fc_esc_stack_20x20mm (Autodesk Fusion 360 design; units mm, degrees)
Autodesk Fusion 360 part; units mm, degrees
sketch "Sketch1" plane through (0, 0, 0) normal (0, 1, 0) x (1, 0, 0)
  line L0 (13.5, -13.5) -> (-13.5, -13.5)
  line L1 (-13.5, -13.5) -> (-13.5, 13.5)
  line L2 (-13.5, 13.5) -> (13.5, 13.5)
  line L3 (13.5, 13.5) -> (13.5, -13.5)
  line L4 (13.5, -13.5) -> (-13.5, 13.5) construction
  line L5 (-13.5, -13.5) -> (13.5, 13.5) construction
  circle A0 centre (10, -10) radius 1.5
  circle A1 centre (-10, -10) radius 1.5
  circle A2 centre (-10, 10) radius 1.5
  circle A3 centre (10, 10) radius 1.5
  line L6 (10, 10) -> (-10, 10) construction
  line L7 (-10, 10) -> (-10, -10) construction
  line L8 (-10, -10) -> (10, -10) construction
  line L9 (10, -10) -> (10, 10) construction
  line L10 (10, 10) -> (-10, -10) construction
  line L11 (-10, 10) -> (10, -10) construction
  circle A4 centre (-10, 10) radius 2.25
  circle A5 centre (10, 10) radius 2.25
  circle A6 centre (10, -10) radius 2.25
  circle A7 centre (-10, -10) radius 2.25
  line L12 (13.5, 11) -> (15.5, 11)
  line L13 (15.5, 11) -> (15.5, 9)
  line L14 (15.5, 9) -> (13.5, 9)
  line L15 (13.5, 7) -> (15.5, 7)
  line L16 (15.5, 7) -> (15.5, 5)
  line L17 (15.5, 5) -> (13.5, 5)
  line L18 (13.5, 3) -> (15.5, 3)
  line L19 (15.5, 3) -> (15.5, 1)
  line L20 (15.5, 1) -> (13.5, 1)
  line L21 (0, 13.5) -> (0, -13.5) construction
  line L22 (13.5, 0) -> (-13.5, 0) construction
  line L23 (15.5, -3) -> (15.5, -1)
  line L24 (15.5, -1) -> (13.5, -1)
  line L25 (13.5, -3) -> (15.5, -3)
  line L26 (15.5, -7) -> (15.5, -5)
  line L27 (15.5, -5) -> (13.5, -5)
  line L28 (13.5, -7) -> (15.5, -7)
  line L29 (15.5, -11) -> (15.5, -9)
  line L30 (15.5, -9) -> (13.5, -9)
  line L31 (13.5, -11) -> (15.5, -11)
  line L32 (-15.5, -11) -> (-15.5, -9)
  line L33 (-15.5, -9) -> (-13.5, -9)
  line L34 (-13.5, -11) -> (-15.5, -11)
  line L35 (-15.5, -7) -> (-15.5, -5)
  line L36 (-15.5, -5) -> (-13.5, -5)
  line L37 (-13.5, -7) -> (-15.5, -7)
  line L38 (-15.5, -3) -> (-15.5, -1)
  line L39 (-15.5, -1) -> (-13.5, -1)
  line L40 (-13.5, -3) -> (-15.5, -3)
  line L41 (-13.5, 3) -> (-15.5, 3)
  line L42 (-15.5, 3) -> (-15.5, 1)
  line L43 (-15.5, 1) -> (-13.5, 1)
  line L44 (-13.5, 7) -> (-15.5, 7)
  line L45 (-15.5, 7) -> (-15.5, 5)
  line L46 (-15.5, 5) -> (-13.5, 5)
  line L47 (-13.5, 11) -> (-15.5, 11)
  line L48 (-15.5, 11) -> (-15.5, 9)
  line L49 (-15.5, 9) -> (-13.5, 9)
  dimension "d1287" = 27
  dimension "d1288" = 27
  dimension "d1292" = 3
  dimension "d1293" = 3
  dimension "d1294" = 3
  dimension "d1295" = 3
  dimension "d1300" = 0
  dimension "d1301" = 0
  dimension "d1302" = 0
  dimension "d1303" = 0
  dimension "d1312" = 20
  dimension "d1313" = 20
  dimension "d1" = 4.5
  dimension "d2" = 4.5
  dimension "d3" = 4.5
  dimension "d4" = 4.5
  dimension "d16" = 10
  dimension "d17" = 2
  dimension "d18" = 2
  dimension "d20" = 1
  dimension "d21" = 31
  measures "d1287" distance of L1 L3
  measures "d1288" distance of L0 L2
  measures "d1292" diameter of A0
  measures "d1293" diameter of A1
  measures "d1294" diameter of A2
  measures "d1295" diameter of A3
  measures "d1312" distance of A1.centre A0.centre
  measures "d1313" distance of A2.centre A1.centre
  measures "d1" diameter of A4
  measures "d2" diameter of A5
  measures "d3" diameter of A6
  measures "d4" diameter of A7
  measures "d16" distance of L12 L20
  measures "d17" distance of L17 L18
  measures "d18" distance of L14 L15
  measures "d20" distance of L20 L22.start
  measures "d21" distance of L13 L48
extrude "Extrude4" add sketch "Sketch1" along normal blind 12 and the other way blind 3 contours A4 | A5 | A6 | A7 makes body 1 at (-7.7528, 8, 10.1122) makes body 2 at (12.2472, 8, 10.1122) makes body 3 at (-7.7528, 8, -9.8878) makes body 4 at (12.2472, 8, -9.8878)
extrude "Extrude3" add sketch "Sketch1" along normal blind 4 contours L0 L1 L2 L3 | A4 | A5 | A6 | A7 bodies 1 2 3 4
extrude "Extrude6" add sketch "Sketch1" along normal blind 2 and the other way blind -0.5 contours L3 L29 L30 L31 | L1 L32 L33 L34 | L3 L26 L27 L28 | L1 L35 L36 L37 | L3 L23 L24 L25 | L1 L38 L39 L40 | L3 L18 L19 L20 | L1 L41 L42 L43 | L3 L15 L16 L17 | L1 L44 L45 L46 | L3 L12 L13 L14 | L1 L47 L48 L49 bodies 1
sketch "Sketch2" plane through (0, 12, 0) normal (0, 1, 0) x (-1, 0, 0)
  circle A0 centre (10, 10) radius 1.5
  circle A1 centre (10, 10) radius 2.25
  circle A2 centre (-10, -10) radius 2.25
  circle A3 centre (-10, 10) radius 2.25
  circle A4 centre (10, 10) radius 2.25
  circle A5 centre (10, -10) radius 2.25
  line L0 (13.5, -13.5) -> (-13.5, -13.5)
  line L1 (-13.5, -13.5) -> (-13.5, 13.5)
  line L2 (-13.5, 13.5) -> (13.5, 13.5)
  line L3 (13.5, 13.5) -> (13.5, -13.5)
  line L4 (-13.5, 13.5) -> (13.5, -13.5) construction
  dimension "d9" = 27
  dimension "d10" = 27
  measures "d9" distance of L0.start L0.end
  measures "d10" distance of L0.start L2.end
extrude "Extrude5" add sketch "Sketch2" against normal blind 4 contours A0 | A1 A4 | A2 | A3 | A5 | L0 L1 L2 L3 bodies 1
chamfer "Chamfer1" distance 1.6 angle 45 4 edges at (13.5, 10, -13.5) (-13.5, 10, -13.5) (-13.5, 10, 13.5) (13.5, 10, 13.5) on bodies 1
fillet "Fillet1" radius 3.4 4 edges at (13.5, 2, 13.5) (13.5, 2, -13.5) (-13.5, 2, -13.5) (-13.5, 2, 13.5) on bodies 1
